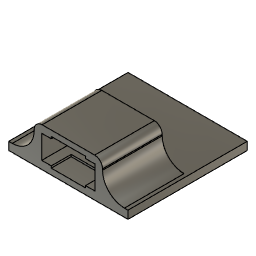
USB A Female Housing (Autodesk Fusion 360 design; units mm, degrees)
Autodesk Fusion 360 part; units mm, degrees
sketch "Sketch1" plane through (0, 0, 0) normal (0, 1, 0) x (1, 0, 0)
  line L0 (6.6, -2.9) -> (-6.6, -2.9)
  line L1 (-6.6, -2.9) -> (-6.6, 2.9)
  line L2 (-6.6, 2.9) -> (6.6, 2.9)
  line L3 (6.6, 2.9) -> (6.6, -2.9)
  line L4 (6.6, -2.9) -> (-6.6, 2.9) construction
  line L5 (-6.6, -2.9) -> (6.6, 2.9) construction
  line L6 (15, 2.9) -> (-15, 2.9)
  line L7 (-15, 2.9) -> (-15, 4.9)
  line L8 (-15, 4.9) -> (15, 4.9)
  line L9 (15, 4.9) -> (15, 2.9)
  line L10 (15, 2.9) -> (-15, 4.9) construction
  line L11 (-15, 2.9) -> (15, 4.9) construction
  line L12 (-8.6, 4.9) -> (8.6, 4.9)
  line L13 (8.6, 4.9) -> (8.6, -4.9)
  line L14 (8.6, -4.9) -> (-8.6, -4.9)
  line L15 (-8.6, -4.9) -> (-8.6, 4.9)
  line L16 (-6.7, 3) -> (6.7, 3)
  line L17 (6.7, 3) -> (6.7, -3)
  line L18 (6.7, -3) -> (-6.7, -3)
  line L19 (-6.7, -3) -> (-6.7, 3)
  line L20 (0, 0) -> (-2.8, 0)
  line L21 (0, 0) -> (2.8, 0)
  line L22 (-1.3, -3.5) -> (-4.3, -3.5)
  line L23 (-4.3, -3.5) -> (-4.3, 3.5)
  line L24 (-4.3, 3.5) -> (-1.3, 3.5)
  line L25 (-1.3, 3.5) -> (-1.3, -3.5)
  line L26 (-1.3, -3.5) -> (-4.3, 3.5) construction
  line L27 (-4.3, -3.5) -> (-1.3, 3.5) construction
  line L28 (4.3, -3.5) -> (1.3, -3.5)
  line L29 (1.3, -3.5) -> (1.3, 3.5)
  line L30 (1.3, 3.5) -> (4.3, 3.5)
  line L31 (4.3, 3.5) -> (4.3, -3.5)
  line L32 (4.3, -3.5) -> (1.3, 3.5) construction
  line L33 (1.3, -3.5) -> (4.3, 3.5) construction
  line L34 (-4.3, 3.5) -> (4.7, 3.5)
  line L35 (4.7, 3.5) -> (4.7, 3.4)
  line L36 (4.7, 3.4) -> (-4.3, 3.4)
  line L37 (-4.3, 3.4) -> (-4.3, 3.5)
  line L38 (-1.3, -3.5) -> (1.3, -3.5)
  line L39 (0, 3) -> (0, -0.7)
  line L40 (-3.75, -0.7) -> (3.75, -0.7)
  line L41 (3.75, -0.7) -> (3.75, 3)
  line L42 (3.75, 3) -> (-3.75, 3)
  line L43 (-3.75, 3) -> (-3.75, -0.7)
  line L44 (-3.75, -0.7) -> (3.75, 3) construction
  line L45 (3.75, -0.7) -> (-3.75, 3) construction
  point P0 (0, 3.9)
  point P1 (-2.8, 0)
  point P2 (2.8, 0)
  point P3 (0, 1.15)
  dimension "d1" = 13.2
  dimension "d2" = 5.8
  dimension "d4" = 30
  dimension "d5" = 2
  dimension "d6" = -2
  dimension "d15" = -0.1
  dimension "d16" = 2.8
  dimension "d17" = 2.8
  dimension "d18" = 3
  dimension "d19" = 7
  dimension "d20" = 3
  dimension "d21" = 7
  dimension "d22" = 9
  dimension "d23" = 0.1
  dimension "d26" = 3.7
  dimension "d27" = 7.5
  dimension "d28" = 3.7
  constraint horizontal L0
  constraint perpendicular L0 L1
  constraint parallel L0 L2
  constraint parallel L1 L3
  constraint coincident L4 L20.start
  constraint coincident L5 L20.start
  constraint coincident L20.start L21.start
  constraint horizontal L6
  constraint perpendicular L6 L7
  constraint parallel L6 L8
  constraint parallel L7 L9
  constraint coincident L10 P0
  constraint coincident L11 P0
  constraint horizontal L20
  constraint parallel L20 L21
  constraint horizontal L22
  constraint perpendicular L22 L23
  constraint parallel L22 L24
  constraint parallel L23 L25
  constraint coincident L26 P1
  constraint coincident L27 P1
  constraint coincident P1 L20.end
  constraint horizontal L28
  constraint perpendicular L28 L29
  constraint parallel L28 L30
  constraint parallel L29 L31
  constraint coincident L32 P2
  constraint coincident L33 P2
  constraint coincident P2 L21.end
  constraint horizontal L34
  constraint vertical L35
  constraint horizontal L36
  constraint vertical L37
  constraint midpoint L16 L39.start
  constraint perpendicular L2 L39
  constraint horizontal L40
  constraint perpendicular L40 L41
  constraint parallel L40 L42
  constraint parallel L41 L43
  constraint coincident L44 P3
  constraint coincident L45 P3
  constraint midpoint L39 P3
  measures "d1" distance of L1.end L2.end
  measures "d2" distance of L0.end L1.end
  measures "d4" distance of L7.end L8.end
  measures "d5" distance of L6.end L7.end
  measures "d16" distance of L20.start P1
  measures "d17" distance of L20.start P2
  measures "d18" distance of L23.end L24.end
  measures "d19" distance of L22.end L23.end
  measures "d20" distance of L29.end L30.end
  measures "d21" distance of L28.end L29.end
  measures "d22" distance of L23.end L34.end
  measures "d23" distance of L23.end L36.end
  measures "d26" distance of L39.start L39.end
  measures "d27" distance of L41.end L42.end
  measures "d28" distance of L40.end L41.end
extrude "Extrude1" add sketch "Sketch1" along normal blind 30 contours L2 L6 L16 L17 L31 | L2 L6 L16 L31 L41 | L6 L8 L12 L13 L15 L16 L17 L19 L23 L24 L30 L31 L34 L35 L36 L37 | L2 L6 L16 L29 L41 L42 | L16 L29 L31 L36 L42 | L6 L8 L9 L13 | L2 L6 L16 L29 L39 L42 | L29 L30 L31 L34 L36 | L31 L34 L35 L36 | L2 L6 L16 L23 L43 | L2 L6 L16 L19 L23 | L2 L6 L16 L25 L39 L42 | L16 L25 L29 L36 L42 | L25 L29 L34 L36 | L6 L7 L8 L15 | L2 L6 L16 L25 L42 L43 | L16 L23 L25 L36 L42 | L23 L24 L25 L34 L36 L37
extrude "Extrude2" add sketch "Sketch1" along normal blind 15 contours L18 L28 L29 L31 | L6 L13 L14 L15 L17 L18 L19 L22 L23 L28 L31 L38 | L18 L25 L29 L38 | L18 L22 L23 L25
fillet "Fillet1" radius 5.5 2 edges at (-8.6, 7.5, -2.9) (8.6, 7.5, -2.9)
fillet "Fillet1" radius 2 2 edges at (-8.6, 7.5, 4.9) (8.6, 7.5, 4.9)
extrude "Extrude3" cut sketch "Sketch1" along normal blind 5 contours L2 L6 L16 L31 L41 | L18 L28 L29 L31 | L18 L25 L29 L38 | L2 L6 L16 L29 L41 L42 | L16 L29 L31 L36 L42 | L18 L22 L23 L25 | L2 L6 L16 L29 L39 L42 | L2 L6 L16 L23 L43 | L2 L6 L16 L25 L39 L42 | L16 L25 L29 L36 L42 | L2 L6 L16 L25 L42 L43 | L16 L23 L25 L36 L42
